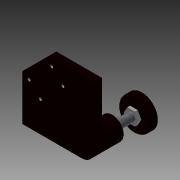
# Autodesk Inventor part: foot
Saved by Autodesk Inventor 2015 (Build 190159000, 159)
## iProperties
Created: 2015-12-24
Part Number: foot
Material: 一般
Document SubType Name: Modeling
Designer: Ryo
Density: 1 g/cm^3
Appearance: 既定
Author: Ryo
Autodesk Inventor part; units mm, degrees
ref_plane "YZ Plane" through (0, 0, 0) normal (1, 0, 0) x (0, 1, 0)
ref_plane "XZ Plane" through (0, 0, 0) normal (0, 1, 0) x (-1, 0, 0)
ref_plane "XY Plane" through (0, 0, 0) normal (0, 0, 1) x (1, 0, 0)
sketch "スケッチ1" plane through (0, 0, 0) normal (0, 1, 0) x (-1, 0, 0)
  line L0 (62.5, -62.5) -> (-42.5, -62.5)
  line L1 (-62.5, -42.5) -> (-62.5, 62.5)
  line L2 (-62.5, 62.5) -> (62.5, 62.5)
  line L3 (62.5, 62.5) -> (62.5, -62.5)
  line L4 (62.5, -62.5) -> (-62.5, 62.5) construction
  line L5 (-62.5, -62.5) -> (62.5, 62.5) construction
  line L6 (17.5, 62.5) -> (62.5, 17.5)
  circle A0 centre (-42.5, -42.5) radius 20
  point P0 (0, 0)
  dimension "d0" = 125
  dimension "d1" = 125
  dimension "d2" = 80
  dimension "d3" = 80
  dimension "d4" = 40
  dimension "d5" = 20
  constraints: 14 end point, 3 point on line, 2 midpoint, 2 parallel, 2 point on circle, 1 centre point, 1 horizontal, 1 perpendicular
  measures "d0" distance of L1.end L2.end
  measures "d1" distance of L5.start L1.end
  measures "d2" distance from line of L6.start L1
  measures "d3" distance from line of L6.end L0
  measures "d4" diameter of A0
  measures "d5" distance from line of L1 A0.centre
extrude "押し出し1" add sketch "スケッチ1" along normal blind 15 contours L0 A0 L1 L2 L6 L3
extrude "押し出し2" add sketch "スケッチ1" along normal blind 53 contours A0
sketch "スケッチ2" plane through (42.5, 53, -42.5) normal (0, 1, 0) x (1, 0, 0)
  point P0 (-42.5, -42.5)
sketch "スケッチ3" plane through (42.5, 53, -42.5) normal (0, 1, 0) x (1, 0, 0)
  circle A0 centre (0, 0) radius 20 projected
  circle A1 centre (0, 0) radius 7.5
  line L0 (13.1788, 0) -> (6.5894, -11.4132)
  line L1 (6.5894, -11.4132) -> (-6.5894, -11.4132)
  line L2 (-6.5894, -11.4132) -> (-13.1788, 0)
  line L3 (-13.1788, 0) -> (-6.5894, 11.4132)
  line L4 (-6.5894, 11.4132) -> (6.5894, 11.4132)
  line L5 (6.5894, 11.4132) -> (13.1788, 0)
  point P0 (-42.5, -42.5)
  dimension "d10" = 15
  constraints: 12 end point, 2 coincident, 1 centre point, 13 other
  measures "d10" diameter of A1
extrude "押し出し3" add sketch "スケッチ3" along normal blind 38 contours A1
extrude "押し出し4" add sketch "スケッチ3" along normal blind 5 contours L0 L1 L2 L3 L4 L5
sketch "スケッチ4" plane through (42.5, 91, -42.5) normal (0, 1, 0) x (1, 0, 0)
  circle A0 centre (0, 0) radius 7.5 projected
  line L0 (6.5894, -11.4132) -> (13.1788, 0) projected
  line L1 (13.1788, 0) -> (6.5894, 11.4132) projected
  line L2 (6.5894, 11.4132) -> (-6.5894, 11.4132) projected
  line L3 (-6.5894, 11.4132) -> (-13.1788, 0) projected
  line L4 (-13.1788, 0) -> (-6.5894, -11.4132) projected
  line L5 (-6.5894, -11.4132) -> (6.5894, -11.4132) projected
  circle A1 centre (0, 0) radius 7.5 projected
  point P0 (-42.5, -42.5)
extrude "押し出し5" add sketch "スケッチ4" against normal blind 5
thread "ねじ1" size "M15x1.5" class "6g" standard "ANSI Metric M Profile" full length
sketch "スケッチ5" plane through (42.5, 91, -42.5) normal (0, 1, 0) x (1, 0, 0)
  circle A0 centre (0, 0) radius 28
  point P0 (-42.5, -42.5)
  dimension "d19" = 56
  constraints: 1 centre point
  measures "d19" diameter of A0
extrude "押し出し6" add sketch "スケッチ5" along normal blind 14
fillet "フィレット1" radius 4 1 edges at (14.5, 91, -42.5)
sketch "スケッチ7" plane through (0, 0, 0) normal (0, -1, 0) x (1, 0, 0)
  point P0 (0, 0)
sketch "スケッチ8" plane through (0, 0, 0) normal (0, -1, 0) x (1, 0, 0)
  circle A0 centre (-50.4462, 10.8482) radius 2.5
  line L0 (62.5, -62.5) -> (-62.5, 62.5) construction
  circle A1 centre (-10.8482, 50.4462) radius 2.5
  circle A2 centre (-30.6472, -8.9508) radius 2.5
  line L1 (-50.4462, 10.8482) -> (-10.8482, 50.4462)
  circle A3 centre (8.9508, 30.6472) radius 2.5
  line L2 (-30.6472, -8.9508) -> (8.9508, 30.6472)
  point P0 (0, 0)
  dimension "d23" = 5
  dimension "d24" = 28
  dimension "d25" = 5
  dimension "d26" = 28
  dimension "d27" = 28
  constraints: 4 centre point, 4 end point, 2 symmetric about line, 2 other
  measures "d23" diameter of A0
  measures "d24" distance from line of L0 L1.start
  measures "d25" diameter of A2
  measures "d26" distance from line of L0 L2.start
  measures "d27" distance between parallel lines of L1 L2
extrude "押し出し7" cut sketch "スケッチ8" against normal blind 15
